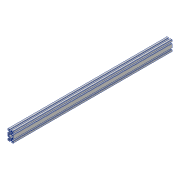
# Autodesk Inventor part: HFS5-2040-300
Saved by Autodesk Inventor 2018 (Build 220112000, 112)
## iProperties
Created: 2018-01-07
Part Number: HFS5-2040-300
Material: Aluminum 6061
Document SubType Name: Modeling
Designer: sawaiz
Density: 2.7 g/cm^3
Appearance: Aluminum - Flat
Author: sawaiz
Autodesk Inventor part; units mm, degrees
ref_plane "YZ Plane" through (0, 0, 0) normal (1, 0, 0) x (0, 1, 0)
ref_plane "XZ Plane" through (0, 0, 0) normal (0, 1, 0) x (-1, 0, 0)
ref_plane "XY Plane" through (0, 0, 0) normal (0, 0, 1) x (1, 0, 0)
sketch "Sketch1" plane through (0, 0, 0) normal (0, 1, 0) x (-1, 0, 0)
  line L0 (-10, 7) -> (-10, -7)
  line L1 (-10, -7) -> (-8, -7)
  line L2 (-8, -7) -> (-8, -4)
  line L3 (-8, -4) -> (-7.0607, -4)
  line L4 (-7.0607, -4) -> (-4, -7.0607)
  line L5 (-4, -7.0607) -> (-4, -7.5)
  line L6 (-4, -7.5) -> (-3.751, -8.7811)
  line L7 (-3.751, -8.7811) -> (-3.933, -9.0964)
  arc A0 (-3.933, -9.0964) -> (-3.933, -9.5964) centre (-3.5, -9.3464) ccw
  line L8 (-3.933, -9.5964) -> (-3.7, -10)
  line L9 (-3.7, -10) -> (-3.933, -10.4036)
  arc A1 (-3.933, -10.4036) -> (-4, -10.6536) centre (-3.5, -10.6536) ccw
  line L10 (-4, -10.6536) -> (-4, -12.9393)
  line L11 (-4, -12.9393) -> (-7.0607, -16)
  line L12 (-7.0607, -16) -> (-8, -16)
  line L13 (-8, -16) -> (-8, -13)
  line L14 (-8, -13) -> (-10, -13)
  line L15 (-10, -13) -> (-10, -19)
  arc A2 (-10, -19) -> (-9, -20) centre (-9, -19) ccw
  line L16 (-9, -20) -> (-3, -20)
  line L17 (-3, -20) -> (-3, -18)
  line L18 (-3, -18) -> (-6, -18)
  line L19 (-6, -18) -> (-6, -17.0607)
  line L20 (-6, -17.0607) -> (-2.9393, -14)
  line L21 (-2.9393, -14) -> (-2.5, -14)
  line L22 (-2.5, -14) -> (-1.2189, -13.751)
  line L23 (-1.2189, -13.751) -> (-0.9036, -13.933)
  arc A3 (-0.9036, -13.933) -> (-0.4036, -13.933) centre (-0.6536, -13.5) ccw
  line L24 (-0.4036, -13.933) -> (0, -13.7)
  line L25 (0, -13.7) -> (0.4036, -13.933)
  arc A4 (0.4036, -13.933) -> (0.6536, -14) centre (0.6536, -13.5) ccw
  line L26 (0.6536, -14) -> (2.9393, -14)
  line L27 (2.9393, -14) -> (6, -17.0607)
  line L28 (6, -17.0607) -> (6, -18)
  line L29 (6, -18) -> (3, -18)
  line L30 (3, -18) -> (3, -20)
  line L31 (3, -20) -> (9, -20)
  arc A5 (9, -20) -> (10, -19) centre (9, -19) ccw
  line L32 (10, -19) -> (10, -13)
  line L33 (10, -13) -> (8, -13)
  line L34 (8, -13) -> (8, -16)
  line L35 (8, -16) -> (7.0607, -16)
  line L36 (7.0607, -16) -> (4, -12.9393)
  line L37 (4, -12.9393) -> (4, -12.5)
  line L38 (4, -12.5) -> (3.751, -11.2189)
  line L39 (3.751, -11.2189) -> (3.933, -10.9036)
  arc A6 (3.933, -10.9036) -> (3.933, -10.4036) centre (3.5, -10.6536) ccw
  line L40 (3.933, -10.4036) -> (3.7, -10)
  line L41 (3.7, -10) -> (3.933, -9.5964)
  arc A7 (3.933, -9.5964) -> (4, -9.3464) centre (3.5, -9.3464) ccw
  line L42 (4, -9.3464) -> (4, -7.0607)
  line L43 (4, -7.0607) -> (7.0607, -4)
  line L44 (7.0607, -4) -> (8, -4)
  line L45 (8, -4) -> (8, -7)
  line L46 (8, -7) -> (10, -7)
  line L47 (10, -7) -> (10, 7)
  line L48 (10, 7) -> (8, 7)
  line L49 (8, 7) -> (8, 4)
  line L50 (8, 4) -> (7.0607, 4)
  line L51 (7.0607, 4) -> (4, 7.0607)
  line L52 (4, 7.0607) -> (4, 9.3464)
  arc A8 (4, 9.3464) -> (3.933, 9.5964) centre (3.5, 9.3464) ccw
  line L53 (3.933, 9.5964) -> (3.7, 10)
  line L54 (3.7, 10) -> (3.933, 10.4036)
  arc A9 (3.933, 10.4036) -> (3.933, 10.9036) centre (3.5, 10.6536) ccw
  line L55 (3.933, 10.9036) -> (3.751, 11.2189)
  line L56 (3.751, 11.2189) -> (4, 12.5)
  line L57 (4, 12.5) -> (4, 12.9393)
  line L58 (4, 12.9393) -> (7.0607, 16)
  line L59 (7.0607, 16) -> (8, 16)
  line L60 (8, 16) -> (8, 13)
  line L61 (8, 13) -> (10, 13)
  line L62 (10, 13) -> (10, 19)
  arc A10 (10, 19) -> (9, 20) centre (9, 19) ccw
  line L63 (9, 20) -> (3, 20)
  line L64 (3, 20) -> (3, 18)
  line L65 (3, 18) -> (6, 18)
  line L66 (6, 18) -> (6, 17.0607)
  line L67 (6, 17.0607) -> (2.9393, 14)
  line L68 (2.9393, 14) -> (0.6536, 14)
  arc A11 (0.6536, 14) -> (0.4036, 13.933) centre (0.6536, 13.5) ccw
  line L69 (0.4036, 13.933) -> (0, 13.7)
  line L70 (0, 13.7) -> (-0.4036, 13.933)
  arc A12 (-0.4036, 13.933) -> (-0.9036, 13.933) centre (-0.6536, 13.5) ccw
  line L71 (-0.9036, 13.933) -> (-1.2189, 13.751)
  line L72 (-1.2189, 13.751) -> (-2.5, 14)
  line L73 (-2.5, 14) -> (-2.9393, 14)
  line L74 (-2.9393, 14) -> (-6, 17.0607)
  line L75 (-6, 17.0607) -> (-6, 18)
  line L76 (-6, 18) -> (-3, 18)
  line L77 (-3, 18) -> (-3, 20)
  line L78 (-3, 20) -> (-9, 20)
  arc A13 (-9, 20) -> (-10, 19) centre (-9, 19) ccw
  line L79 (-10, 19) -> (-10, 13)
  line L80 (-10, 13) -> (-8, 13)
  line L81 (-8, 13) -> (-8, 16)
  line L82 (-8, 16) -> (-7.0607, 16)
  line L83 (-7.0607, 16) -> (-4, 12.9393)
  line L84 (-4, 12.9393) -> (-4, 10.6536)
  arc A14 (-4, 10.6536) -> (-3.933, 10.4036) centre (-3.5, 10.6536) ccw
  line L85 (-3.933, 10.4036) -> (-3.7, 10)
  line L86 (-3.7, 10) -> (-3.933, 9.5964)
  arc A15 (-3.933, 9.5964) -> (-3.933, 9.0964) centre (-3.5, 9.3464) ccw
  line L87 (-3.933, 9.0964) -> (-3.751, 8.7811)
  line L88 (-3.751, 8.7811) -> (-4, 7.5)
  line L89 (-4, 7.5) -> (-4, 7.0607)
  line L90 (-4, 7.0607) -> (-7.0607, 4)
  line L91 (-7.0607, 4) -> (-8, 4)
  line L92 (-8, 4) -> (-8, 7)
  arc A16 (-7.7, 2) -> (-8, 1.7) centre (-7.7, 1.7) ccw
  line L93 (-7.0636, 2) -> (-7.7, 2)
  arc A17 (-7.0636, 2) -> (-6.8515, 2.0879) centre (-7.0636, 2.3) ccw
  line L94 (-2.9393, 6) -> (-6.8515, 2.0879)
  line L95 (2.9393, 6) -> (-2.9393, 6)
  line L96 (6.8515, 2.0879) -> (2.9393, 6)
  arc A18 (6.8515, 2.0879) -> (7.0636, 2) centre (7.0636, 2.3) ccw
  line L97 (7.7, 2) -> (7.0636, 2)
  arc A19 (8, 1.7) -> (7.7, 2) centre (7.7, 1.7) ccw
  line L98 (8, -1.7) -> (8, 1.7)
  arc A20 (7.7, -2) -> (8, -1.7) centre (7.7, -1.7) ccw
  line L99 (7.0636, -2) -> (7.7, -2)
  arc A21 (7.0636, -2) -> (6.8515, -2.0879) centre (7.0636, -2.3) ccw
  line L100 (2.9393, -6) -> (6.8515, -2.0879)
  line L101 (-2.9393, -6) -> (2.9393, -6)
  line L102 (-6.8515, -2.0879) -> (-2.9393, -6)
  arc A22 (-6.8515, -2.0879) -> (-7.0636, -2) centre (-7.0636, -2.3) ccw
  line L103 (-7.7, -2) -> (-7.0636, -2)
  arc A23 (-8, -1.7) -> (-7.7, -2) centre (-7.7, -1.7) ccw
  line L104 (-8, 1.7) -> (-8, -1.7)
  line L105 (-8, 7) -> (-10, 7)
  circle A24 centre (0, 10) radius 2.1
  circle A25 centre (0, -10) radius 2.1
  line L106 (0, -10) -> (0, 10) construction
  point P0 (0, 0)
  point P1 (0, 0)
  constraints: 214 end point, 48 point on circle, 26 centre point, 1 coincident, 1 midpoint, 1 vertical
extrude "Extrusion1" add sketch "Sketch1" along normal mid plane 600
body "Solid1"
